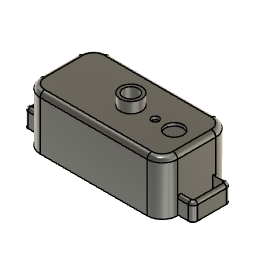
EnclosureTop with Ext Mic Aperture (Autodesk Fusion 360 design; units mm, degrees)
Autodesk Fusion 360 part; units mm, degrees
box "BoxPrimitive2" add length 35 width 90 height 45 placed x (0, 0, 1) y (1, 0, 0) z (0, 1, 0) at (15, 0, 0) makes body 1
fillet "Fillet1" radius 10 1 edges at (15, 0, 17.5) on bodies 1
fillet "Fillet2" radius 10 1 edges at (105, 0, 17.5) on bodies 1
fillet "Fillet3" radius 10 1 edges at (15, 45, 17.5) on bodies 1
fillet "Fillet4" radius 10 1 edges at (105, 45, 17.5) on bodies 1
fillet "Fillet5" radius 3 8 edges at (102.0711, 2.9289, 35) (60, 0, 35) (17.9289, 2.9289, 35) (15, 22.5, 35) (17.9289, 42.0711, 35) (60, 45, 35) (102.0711, 42.0711, 35) (105, 22.5, 35) 1 faces at (48.3333, 15, 35) on bodies 1
shell "Shell1" thickness 2 removed faces 1 at (48.3333, 15, 0) on bodies 1
cylinder "CylinderPrimitive1" add diameter 14 height 7 placed x (1, 0, 0) y (0, 1, 0) z (0, 0, 1) at (62, 23, 35) bodies 1
hole "Hole1" at (62.0207, 22.9694, 42) direction (0, 0, -1) diameter 10 depth 14 tip angle 180 bodies 1
hole "Hole2" at (90.2018, 22.554, 35) direction (0, 0, -1) diameter 11.8 depth 3 tip angle 180 bodies 1
hole "Hole3" at (77.8978, 22.4863, 35) direction (0, 0, -1) diameter 4.8 depth 3 tip angle 180 bodies 1
move_face "MoveFace1" by (0, -1, 0) 1 faces at (58.4466, 28.2119, 42) on bodies 1
move_face "MoveFace2" by (0, -0.6049, 0) 1 faces at (58.4466, 28.2119, 42) on bodies 1
move_body "Move1" bodies 1 to x (1, 0, 0) y (0, 1, 0) z (0, 0, 1) at (0.2745, 3.7742, 0)
move_face "MoveFace3" by (0, -1, 0) 1 faces at (58.721, 31.986, 42) on bodies 1
move_face "MoveFace4" by (0, -1.6862, 0) 1 faces at (58.721, 31.986, 42) on bodies 1
move_face "MoveFace5" by (0, -1, 0) 1 faces at (58.721, 31.986, 42) on bodies 1
move_face "MoveFace6" by (0, -0.6176, 0) 1 faces at (58.721, 31.986, 42) on bodies 1
move_face "MoveFace7" to x (1, 0, 0) y (0, 1, 0) z (0, 0, 1) at (0, -1, 0) 1 faces at (69.2397, 26.0772, 37.3333) on bodies 1
move_face "MoveFace8" to x (1, 0, 0) y (0, 1, 0) z (0, 0, 1) at (0, -1, 0) 1 faces at (62.793, 21.7684, 36) on bodies 1
move_face "MoveFace9" to x (1, 0, 0) y (0, 1, 0) z (0, 0, 1) at (0, 0.4, 0) 1 faces at (69.2397, 26.4712, 37.3333) on bodies 1
move_face "MoveFace10" to x (1, 0, 0) y (0, 1, 0) z (0, 0, 1) at (0, 0.4, 0) 1 faces at (62.793, 20.7684, 36) on bodies 1
cylinder "CylinderPrimitive2" add diameter 10.692 height 10 placed x (0, 1, 0) y (1, 0, 0) z (0, 0, -1) at (25.2745, 38.7742, 33) bodies 1
cylinder "CylinderPrimitive3" add diameter 10 height 10 placed x (0, 1, 0) y (1, 0, 0) z (0, 0, -1) at (25.2745, 13.7742, 33) bodies 1
delete_face "DeleteFace1" 2 faces at (26.1309, 40.8923, 23) (24.7422, 44.0936, 26.3333) on bodies 1
cylinder "CylinderPrimitive4" add diameter 10 height 10 placed x (0, 1, 0) y (1, 0, 0) z (0, 0, -1) at (25.2745, 38.7742, 33) bodies 1
cylinder "CylinderPrimitive5" add diameter 10 height 10 placed x (0, 1, 0) y (1, 0, 0) z (0, 0, -1) at (95.2745, 38.7742, 33) bodies 1
cylinder "CylinderPrimitive6" add diameter 10 height 10 placed x (0, 1, 0) y (1, 0, 0) z (0, 0, -1) at (95.2745, 13.7742, 33) bodies 1
box "BoxPrimitive3" add length 11.656 width 25 height 10 placed x (0, 0, 1) y (0, -1, 0) z (1, 0, 0) at (105.2745, 38.7742, 0) bodies 1
fillet "Fillet6" radius 1 8 edges at (103.2745, 26.2742, 0) (100.9313, 44.431, 0) (60.2745, 46.7742, 0) (19.6176, 44.431, 0) (17.2745, 26.2742, 0) (19.6176, 8.1173, 0) (60.2745, 5.7742, 0) (100.9313, 8.1173, 0) on bodies 1
fillet "Fillet7" radius 0.5 3 edges at (110.2745, 38.7742, 0) (115.2745, 26.2742, 0) (110.2745, 13.7742, 0) on bodies 1
fillet "Fillet8" radius 2 3 edges at (115.2745, 26.2742, 11.656) (110.2745, 38.7742, 11.656) (110.2745, 13.7742, 11.656) on bodies 1
fillet "Fillet9" radius 3 6 edges at (115.128, 38.6277, 0.1464) (115.2745, 38.7742, 5.078) (114.6887, 38.1884, 11.0702) (114.6887, 14.36, 11.0702) (115.2745, 13.7742, 5.078) (115.128, 13.9206, 0.1464) on bodies 1
sketch "Sketch10" plane through (0, 0, 11.656) normal (0, 0, 1) x (-1, 0, 0)
  arc A0 (-112.2745, -15.7742) -> (-113.2745, -16.7742) centre (-112.2745, -16.7742) ccw
  line L0 (-113.2745, -16.7742) -> (-113.2745, -35.7742)
  arc A1 (-113.2745, -35.7742) -> (-112.2745, -36.7742) centre (-112.2745, -35.7742) ccw
  line L1 (-112.2745, -36.7742) -> (-105.2745, -36.7742)
  line L2 (-105.2745, -36.7742) -> (-105.2745, -15.7742)
  line L3 (-105.2745, -15.7742) -> (-112.2745, -15.7742)
  line L4 (-105.2745, -15.7742) -> (-111.7745, -15.7742)
  line L5 (-113.2745, -17.2742) -> (-113.2745, -35.2742)
  line L6 (-111.7745, -36.7742) -> (-105.2745, -36.7742)
  line L7 (-105.2745, -36.7742) -> (-105.2745, -15.7742)
  arc A2 (-111.7745, -15.7742) -> (-113.2745, -17.2742) centre (-111.7745, -17.2742) ccw
  arc A3 (-113.2745, -35.2742) -> (-111.7745, -36.7742) centre (-111.7745, -35.2742) ccw
  point P0 (-113.2745, -15.7742)
  dimension "d56" = 8
  dimension "d57" = 21
  dimension "d58" = 1.5
  dimension "d59" = 1.5
  constraint horizontal L4
  constraint vertical L5
  constraint horizontal L6
  constraint vertical L7
  constraint coincident L2.end L3.start
  constraint coincident P0 L4
  constraint coincident P0 L5
  constraint tangent L4 A2
  constraint tangent L5 A2
  constraint tangent L5 A3
  constraint tangent L6 A3
  measures "d56" distance of L2.end P0
  measures "d57" distance of L2.end L1.end
  measures "d58" radius of A2
  measures "d59" radius of A3
extrude "Extrude1" cut sketch "Sketch10" against normal blind 14 contours L0 L1 L2 L3 L4 L5 L6 L7 A2 A3 bodies 1
box "BoxPrimitive4" cut length 25 width 10 height 12 placed x (0, -1, 0) y (1, 0, 0) z (0, 0, 1) at (5.2781, 38.7635, 0) bodies 1
box "BoxPrimitive5" add length 12 width 10 height 25 placed x (0, 0, -1) y (1, 0, 0) z (0, -1, 0) at (5.2745, 38.7635, 12) separate body makes body 2
sketch "Sketch13" plane through (0, 0, 12) normal (0, 0, 1) x (-1, 0, 0)
  line L0 (-15.2745, -13.7635) -> (-15.2745, -38.7635)
  line L1 (-15.2745, -38.7635) -> (-5.2745, -38.7635)
  line L2 (-5.2745, -38.7635) -> (-5.2745, -13.7635)
  line L3 (-5.2745, -13.7635) -> (-15.2745, -13.7635)
  line L4 (-15.2745, -16.0079) -> (-8.7745, -16.0079)
  line L5 (-7.2745, -17.5079) -> (-7.2745, -35.5079)
  line L6 (-8.7745, -37.0079) -> (-15.2745, -37.0079)
  line L7 (-15.2745, -37.0079) -> (-15.2745, -16.0079)
  arc A0 (-7.2745, -17.5079) -> (-8.7745, -16.0079) centre (-8.7745, -17.5079) ccw
  arc A1 (-8.7745, -37.0079) -> (-7.2745, -35.5079) centre (-8.7745, -35.5079) ccw
  point P0 (-7.2745, -16.0079)
  dimension "d72" = 8
  dimension "d73" = 21
  dimension "d74" = 1.5
  constraint horizontal L4
  constraint vertical L5
  constraint horizontal L6
  constraint vertical L7
  constraint coincident L0 L4.start
  constraint coincident P0 L4
  constraint coincident P0 L5
  constraint tangent L4 A0
  constraint tangent L5 A0
  constraint tangent L5 A1
  constraint tangent L6 A1
  constraint equal A0 A1
  measures "d72" distance of L4.start P0
  measures "d73" distance of L4.start L6.end
  measures "d74" radius of A0
extrude "Extrude2" cut sketch "Sketch13" against normal blind 15 contours L0 L4 L5 L6 L7 A0 A1 bodies 2
fillet "Fillet10" radius 2 5 edges at (10.2745, 13.7635, 12) (10.2745, 38.7635, 12) (5.2745, 13.7635, 6) (5.2745, 38.7635, 6) (5.2745, 26.2635, 12) on bodies 2
fillet "Fillet11" radius 0.5 5 edges at (11.2745, 38.7635, 0) (5.8603, 38.1777, 0) (5.2745, 26.2635, 0) (5.8603, 14.3493, 0) (11.2745, 13.7635, 0) on bodies 2
chamfer "Chamfer1" distance 1 angle 45 5 edges at (12.0245, 37.0079, 0) (7.7138, 36.5685, 0) (7.2745, 26.5079, 0) (7.7138, 16.4472, 0) (12.0245, 16.0079, 0) on bodies 2
chamfer "Chamfer2" distance 1 angle 45 5 edges at (113.2745, 26.2742, 0) (112.8351, 36.3348, 0) (108.5245, 36.7742, 0) (108.5245, 15.7742, 0) (112.8351, 16.2135, 0) on bodies 1
